Autodesk Inventor part; units mm, degrees
(part 2 of 2)
sketch "Skizze1 outline for Extrusion1" plane through (0, 0, 0) normal (0, 1, 0) x (-1, 0, 0)
  line L0 (27.3183, 0.0124) -> (29.62197, 0.0124)
  line L1 (27.3183, 0.0995) -> (27.3183, 0.0124)
  line L2 (27.2706, 0.1948) -> (27.3183, 0.0995)
  line L3 (27.223, 0.2424) -> (27.2706, 0.1948)
  line L4 (27.1278, 0.29) -> (27.223, 0.2424)
  line L5 (26.7468, 0.29) -> (27.1278, 0.29)
  line L6 (26.7468, 0.0124) -> (26.7468, 0.29)
  line L7 (11.5266, 0.0124) -> (26.7468, 0.0124)
  line L8 (10.7766, 0.7624) -> (11.5266, 0.0124)
  line L9 (9.7766, 0.7624) -> (10.7766, 0.7624)
  line L10 (9.7766, 0.0124) -> (9.7766, 0.7624)
  line L11 (8.0266, 0.0124) -> (9.7766, 0.0124)
  line L12 (6.5266, 1.5124) -> (8.0266, 0.0124)
  line L13 (1.5266, 1.5124) -> (6.5266, 1.5124)
  line L14 (1.5266, 10.9594) -> (1.5266, 1.5124)
  line L15 (16.4542, 10.9594) -> (1.5266, 10.9594)
  line L16 (26.5126, 21.0178) -> (16.4542, 10.9594)
  line L17 (31.4402, 21.0178) -> (26.5126, 21.0178)
  line L18 (31.4402, 0.0124) -> (31.4402, 21.0178)
  line L19 (30.44313, 0.0124) -> (31.4402, 0.0124)
  line L20 (30.4135, 0.0519) -> (30.44313, 0.0124)
  line L21 (30.38387, 0.0124) -> (30.4135, 0.0519)
  line L22 (29.68123, 0.0124) -> (30.38387, 0.0124)
  line L23 (29.6516, 0.0519) -> (29.68123, 0.0124)
  line L24 (29.62197, 0.0124) -> (29.6516, 0.0519)
  line L25 (20.0386, 33.4228) -> (0.125, 33.4228)
  line L26 (20.7886, 32.6728) -> (20.0386, 33.4228)
  line L27 (21.7886, 32.6728) -> (20.7886, 32.6728)
  line L28 (21.7886, 33.4228) -> (21.7886, 32.6728)
  line L29 (23.5386, 33.4228) -> (21.7886, 33.4228)
  line L30 (25.0386, 31.9228) -> (23.5386, 33.4228)
  line L31 (30.0386, 31.9228) -> (25.0386, 31.9228)
  line L32 (30.0386, 22.4758) -> (30.0386, 31.9228)
  line L33 (15.111, 22.4758) -> (30.0386, 22.4758)
  line L34 (5.0526, 12.4174) -> (15.111, 22.4758)
  line L35 (0.125, 12.4174) -> (5.0526, 12.4174)
  line L36 (0.125, 33.4228) -> (0.125, 12.4174)
  line L37 (27.2183, 36.5124) -> (29.52197, 36.5124)
  line L38 (27.2183, 36.5995) -> (27.2183, 36.5124)
  line L39 (27.1706, 36.6948) -> (27.2183, 36.5995)
  line L40 (27.123, 36.7424) -> (27.1706, 36.6948)
  line L41 (27.0278, 36.79) -> (27.123, 36.7424)
  line L42 (26.6468, 36.79) -> (27.0278, 36.79)
  line L43 (26.6468, 36.5124) -> (26.6468, 36.79)
  line L44 (11.4266, 36.5124) -> (26.6468, 36.5124)
  line L45 (10.6766, 37.2624) -> (11.4266, 36.5124)
  line L46 (9.6766, 37.2624) -> (10.6766, 37.2624)
  line L47 (9.6766, 36.5124) -> (9.6766, 37.2624)
  line L48 (7.9266, 36.5124) -> (9.6766, 36.5124)
  line L49 (6.4266, 38.0124) -> (7.9266, 36.5124)
  line L50 (1.4266, 38.0124) -> (6.4266, 38.0124)
  line L51 (1.4266, 47.4594) -> (1.4266, 38.0124)
  line L52 (16.3542, 47.4594) -> (1.4266, 47.4594)
  line L53 (26.4126, 57.5178) -> (16.3542, 47.4594)
  line L54 (31.3402, 57.5178) -> (26.4126, 57.5178)
  line L55 (31.3402, 36.5124) -> (31.3402, 57.5178)
  line L56 (30.34313, 36.5124) -> (31.3402, 36.5124)
  line L57 (30.3135, 36.5519) -> (30.34313, 36.5124)
  line L58 (30.28387, 36.5124) -> (30.3135, 36.5519)
  line L59 (29.58123, 36.5124) -> (30.28387, 36.5124)
  line L60 (29.5516, 36.5519) -> (29.58123, 36.5124)
  line L61 (29.52197, 36.5124) -> (29.5516, 36.5519)
  line L62 (19.9386, 69.9228) -> (0.025, 69.9228)
  line L63 (20.6886, 69.1728) -> (19.9386, 69.9228)
  line L64 (21.6886, 69.1728) -> (20.6886, 69.1728)
  line L65 (21.6886, 69.9228) -> (21.6886, 69.1728)
  line L66 (23.4386, 69.9228) -> (21.6886, 69.9228)
  line L67 (24.9386, 68.4228) -> (23.4386, 69.9228)
  line L68 (29.9386, 68.4228) -> (24.9386, 68.4228)
  line L69 (29.9386, 58.9758) -> (29.9386, 68.4228)
  line L70 (15.011, 58.9758) -> (29.9386, 58.9758)
  line L71 (4.9526, 48.9174) -> (15.011, 58.9758)
  line L72 (0.025, 48.9174) -> (4.9526, 48.9174)
  line L73 (0.025, 69.9228) -> (0.025, 48.9174)
  line L74 (53.0152, 69.9374) -> (33.1016, 69.9374)
  line L75 (53.7652, 69.1874) -> (53.0152, 69.9374)
  line L76 (54.7652, 69.1874) -> (53.7652, 69.1874)
  line L77 (54.7652, 69.9374) -> (54.7652, 69.1874)
  line L78 (56.5152, 69.9374) -> (54.7652, 69.9374)
  line L79 (58.0152, 68.4374) -> (56.5152, 69.9374)
  line L80 (63.0152, 68.4374) -> (58.0152, 68.4374)
  line L81 (63.0152, 58.9904) -> (63.0152, 68.4374)
  line L82 (48.0876, 58.9904) -> (63.0152, 58.9904)
  line L83 (38.0292, 48.932) -> (48.0876, 58.9904)
  line L84 (33.1016, 48.932) -> (38.0292, 48.932)
  line L85 (33.1016, 69.9374) -> (33.1016, 48.932)
  line L86 (60.2949, 36.527) -> (62.59857, 36.527)
  line L87 (60.2949, 36.6141) -> (60.2949, 36.527)
  line L88 (60.2472, 36.7094) -> (60.2949, 36.6141)
  line L89 (60.1996, 36.757) -> (60.2472, 36.7094)
  line L90 (60.1044, 36.8046) -> (60.1996, 36.757)
  line L91 (59.7234, 36.8046) -> (60.1044, 36.8046)
  line L92 (59.7234, 36.527) -> (59.7234, 36.8046)
  line L93 (44.5032, 36.527) -> (59.7234, 36.527)
  line L94 (43.7532, 37.277) -> (44.5032, 36.527)
  line L95 (42.7532, 37.277) -> (43.7532, 37.277)
  line L96 (42.7532, 36.527) -> (42.7532, 37.277)
  line L97 (41.0032, 36.527) -> (42.7532, 36.527)
  line L98 (39.5032, 38.027) -> (41.0032, 36.527)
  line L99 (34.5032, 38.027) -> (39.5032, 38.027)
  line L100 (34.5032, 47.474) -> (34.5032, 38.027)
  line L101 (49.4308, 47.474) -> (34.5032, 47.474)
  line L102 (59.4892, 57.5324) -> (49.4308, 47.474)
  line L103 (64.4168, 57.5324) -> (59.4892, 57.5324)
  line L104 (64.4168, 36.527) -> (64.4168, 57.5324)
  line L105 (63.41973, 36.527) -> (64.4168, 36.527)
  line L106 (63.3901, 36.5665) -> (63.41973, 36.527)
  line L107 (63.36047, 36.527) -> (63.3901, 36.5665)
  line L108 (62.65783, 36.527) -> (63.36047, 36.527)
  line L109 (62.6282, 36.5665) -> (62.65783, 36.527)
  line L110 (62.59857, 36.527) -> (62.6282, 36.5665)
  line L111 (53.1152, 33.4374) -> (33.2016, 33.4374)
  line L112 (53.8652, 32.6874) -> (53.1152, 33.4374)
  line L113 (54.8652, 32.6874) -> (53.8652, 32.6874)
  line L114 (54.8652, 33.4374) -> (54.8652, 32.6874)
  line L115 (56.6152, 33.4374) -> (54.8652, 33.4374)
  line L116 (58.1152, 31.9374) -> (56.6152, 33.4374)
  line L117 (63.1152, 31.9374) -> (58.1152, 31.9374)
  line L118 (63.1152, 22.4904) -> (63.1152, 31.9374)
  line L119 (48.1876, 22.4904) -> (63.1152, 22.4904)
  line L120 (38.1292, 12.432) -> (48.1876, 22.4904)
  line L121 (33.2016, 12.432) -> (38.1292, 12.432)
  line L122 (33.2016, 33.4374) -> (33.2016, 12.432)
  line L123 (60.3949, 0.027) -> (62.69857, 0.027)
  line L124 (60.3949, 0.1141) -> (60.3949, 0.027)
  line L125 (60.3472, 0.2094) -> (60.3949, 0.1141)
  line L126 (60.2996, 0.257) -> (60.3472, 0.2094)
  line L127 (60.2044, 0.3046) -> (60.2996, 0.257)
  line L128 (59.8234, 0.3046) -> (60.2044, 0.3046)
  line L129 (59.8234, 0.027) -> (59.8234, 0.3046)
  line L130 (44.6032, 0.027) -> (59.8234, 0.027)
  line L131 (43.8532, 0.777) -> (44.6032, 0.027)
  line L132 (42.8532, 0.777) -> (43.8532, 0.777)
  line L133 (42.8532, 0.027) -> (42.8532, 0.777)
  line L134 (41.1032, 0.027) -> (42.8532, 0.027)
  line L135 (39.6032, 1.527) -> (41.1032, 0.027)
  line L136 (34.6032, 1.527) -> (39.6032, 1.527)
  line L137 (34.6032, 10.974) -> (34.6032, 1.527)
  line L138 (49.5308, 10.974) -> (34.6032, 10.974)
  line L139 (59.5892, 21.0324) -> (49.5308, 10.974)
  line L140 (64.5168, 21.0324) -> (59.5892, 21.0324)
  line L141 (64.5168, 0.027) -> (64.5168, 21.0324)
  line L142 (63.51973, 0.027) -> (64.5168, 0.027)
  line L143 (63.4901, 0.0665) -> (63.51973, 0.027)
  line L144 (63.46047, 0.027) -> (63.4901, 0.0665)
  line L145 (62.75783, 0.027) -> (63.46047, 0.027)
  line L146 (62.7282, 0.0665) -> (62.75783, 0.027)
  line L147 (62.69857, 0.027) -> (62.7282, 0.0665)
  line L148 (94.0699, 0.027) -> (96.37357, 0.027)
  line L149 (94.0699, 0.1141) -> (94.0699, 0.027)
  line L150 (94.0222, 0.2094) -> (94.0699, 0.1141)
  line L151 (93.9746, 0.257) -> (94.0222, 0.2094)
  line L152 (93.8794, 0.3046) -> (93.9746, 0.257)
  line L153 (93.4984, 0.3046) -> (93.8794, 0.3046)
  line L154 (93.4984, 0.027) -> (93.4984, 0.3046)
  line L155 (78.2782, 0.027) -> (93.4984, 0.027)
  line L156 (77.5282, 0.777) -> (78.2782, 0.027)
  line L157 (76.5282, 0.777) -> (77.5282, 0.777)
  line L158 (76.5282, 0.027) -> (76.5282, 0.777)
  line L159 (74.7782, 0.027) -> (76.5282, 0.027)
  line L160 (73.2782, 1.527) -> (74.7782, 0.027)
  line L161 (68.2782, 1.527) -> (73.2782, 1.527)
  line L162 (68.2782, 10.974) -> (68.2782, 1.527)
  line L163 (83.2058, 10.974) -> (68.2782, 10.974)
  line L164 (93.2642, 21.0324) -> (83.2058, 10.974)
  line L165 (98.1918, 21.0324) -> (93.2642, 21.0324)
  line L166 (98.1918, 0.027) -> (98.1918, 21.0324)
  line L167 (97.19473, 0.027) -> (98.1918, 0.027)
  line L168 (97.1651, 0.0665) -> (97.19473, 0.027)
  line L169 (97.13547, 0.027) -> (97.1651, 0.0665)
  line L170 (96.43283, 0.027) -> (97.13547, 0.027)
  line L171 (96.4032, 0.0665) -> (96.43283, 0.027)
  line L172 (96.37357, 0.027) -> (96.4032, 0.0665)
  line L173 (86.7902, 33.4374) -> (66.8766, 33.4374)
  line L174 (87.5402, 32.6874) -> (86.7902, 33.4374)
  line L175 (88.5402, 32.6874) -> (87.5402, 32.6874)
  line L176 (88.5402, 33.4374) -> (88.5402, 32.6874)
  line L177 (90.2902, 33.4374) -> (88.5402, 33.4374)
  line L178 (91.7902, 31.9374) -> (90.2902, 33.4374)
  line L179 (96.7902, 31.9374) -> (91.7902, 31.9374)
  line L180 (96.7902, 22.4904) -> (96.7902, 31.9374)
  line L181 (81.8626, 22.4904) -> (96.7902, 22.4904)
  line L182 (71.8042, 12.432) -> (81.8626, 22.4904)
  line L183 (66.8766, 12.432) -> (71.8042, 12.432)
  line L184 (66.8766, 33.4374) -> (66.8766, 12.432)
  line L185 (93.9699, 36.527) -> (96.27357, 36.527)
  line L186 (93.9699, 36.6141) -> (93.9699, 36.527)
  line L187 (93.9222, 36.7094) -> (93.9699, 36.6141)
  line L188 (93.8746, 36.757) -> (93.9222, 36.7094)
  line L189 (93.7794, 36.8046) -> (93.8746, 36.757)
  line L190 (93.3984, 36.8046) -> (93.7794, 36.8046)
  line L191 (93.3984, 36.527) -> (93.3984, 36.8046)
  line L192 (78.1782, 36.527) -> (93.3984, 36.527)
  line L193 (77.4282, 37.277) -> (78.1782, 36.527)
  line L194 (76.4282, 37.277) -> (77.4282, 37.277)
  line L195 (76.4282, 36.527) -> (76.4282, 37.277)
  line L196 (74.6782, 36.527) -> (76.4282, 36.527)
  line L197 (73.1782, 38.027) -> (74.6782, 36.527)
  line L198 (68.1782, 38.027) -> (73.1782, 38.027)
  line L199 (68.1782, 47.474) -> (68.1782, 38.027)
  line L200 (83.1058, 47.474) -> (68.1782, 47.474)
  line L201 (93.1642, 57.5324) -> (83.1058, 47.474)
  line L202 (98.0918, 57.5324) -> (93.1642, 57.5324)
  line L203 (98.0918, 36.527) -> (98.0918, 57.5324)
  line L204 (97.09473, 36.527) -> (98.0918, 36.527)
  line L205 (97.0651, 36.5665) -> (97.09473, 36.527)
  line L206 (97.03547, 36.527) -> (97.0651, 36.5665)
  line L207 (96.33283, 36.527) -> (97.03547, 36.527)
  line L208 (96.3032, 36.5665) -> (96.33283, 36.527)
  line L209 (96.27357, 36.527) -> (96.3032, 36.5665)
  line L210 (86.6902, 69.9374) -> (66.7766, 69.9374)
  line L211 (87.4402, 69.1874) -> (86.6902, 69.9374)
  line L212 (88.4402, 69.1874) -> (87.4402, 69.1874)
  line L213 (88.4402, 69.9374) -> (88.4402, 69.1874)
  line L214 (90.1902, 69.9374) -> (88.4402, 69.9374)
  line L215 (91.6902, 68.4374) -> (90.1902, 69.9374)
  line L216 (96.6902, 68.4374) -> (91.6902, 68.4374)
  line L217 (96.6902, 58.9904) -> (96.6902, 68.4374)
  line L218 (81.7626, 58.9904) -> (96.6902, 58.9904)
  line L219 (71.7042, 48.932) -> (81.7626, 58.9904)
  line L220 (66.7766, 48.932) -> (71.7042, 48.932)
  line L221 (66.7766, 69.9374) -> (66.7766, 48.932)
  line L222 (119.767, 69.952) -> (99.8532, 69.952)
  line L223 (120.517, 69.202) -> (119.767, 69.952)
  line L224 (121.517, 69.202) -> (120.517, 69.202)
  line L225 (121.517, 69.952) -> (121.517, 69.202)
  line L226 (123.267, 69.952) -> (121.517, 69.952)
  line L227 (124.767, 68.452) -> (123.267, 69.952)
  line L228 (129.767, 68.452) -> (124.767, 68.452)
  line L229 (129.767, 59.005) -> (129.767, 68.452)
  line L230 (114.839, 59.005) -> (129.767, 59.005)
  line L231 (104.781, 48.9466) -> (114.839, 59.005)
  line L232 (99.8532, 48.9466) -> (104.781, 48.9466)
  line L233 (99.8532, 69.952) -> (99.8532, 48.9466)
  line L234 (127.046, 36.5416) -> (129.350349, 36.5416)
  line L235 (127.046, 36.6287) -> (127.046, 36.5416)
  line L236 (126.999, 36.724) -> (127.046, 36.6287)
  line L237 (126.951, 36.7716) -> (126.999, 36.724)
  line L238 (126.856, 36.8192) -> (126.951, 36.7716)
  line L239 (126.475, 36.8192) -> (126.856, 36.8192)
  line L240 (126.475, 36.5416) -> (126.475, 36.8192)
  line L241 (111.255, 36.5416) -> (126.475, 36.5416)
  line L242 (110.505, 37.2916) -> (111.255, 36.5416)
  line L243 (109.505, 37.2916) -> (110.505, 37.2916)
  line L244 (109.505, 36.5416) -> (109.505, 37.2916)
  line L245 (107.755, 36.5416) -> (109.505, 36.5416)
  line L246 (106.255, 38.0416) -> (107.755, 36.5416)
  line L247 (101.255, 38.0416) -> (106.255, 38.0416)
  line L248 (101.255, 47.4886) -> (101.255, 38.0416)
  line L249 (116.182, 47.4886) -> (101.255, 47.4886)
  line L250 (126.241, 57.547) -> (116.182, 47.4886)
  line L251 (131.168, 57.547) -> (126.241, 57.547)
  line L252 (131.168, 36.5416) -> (131.168, 57.547)
  line L253 (130.171651, 36.5416) -> (131.168, 36.5416)
  line L254 (130.142, 36.5811) -> (130.171651, 36.5416)
  line L255 (130.112349, 36.5416) -> (130.142, 36.5811)
  line L256 (129.409651, 36.5416) -> (130.112349, 36.5416)
  line L257 (129.38, 36.5811) -> (129.409651, 36.5416)
  line L258 (129.350349, 36.5416) -> (129.38, 36.5811)
  line L259 (119.867, 33.452) -> (99.9532, 33.452)
  line L260 (120.617, 32.702) -> (119.867, 33.452)
  line L261 (121.617, 32.702) -> (120.617, 32.702)
  line L262 (121.617, 33.452) -> (121.617, 32.702)
  line L263 (123.367, 33.452) -> (121.617, 33.452)
  line L264 (124.867, 31.952) -> (123.367, 33.452)
  line L265 (129.867, 31.952) -> (124.867, 31.952)
  line L266 (129.867, 22.505) -> (129.867, 31.952)
  line L267 (114.939, 22.505) -> (129.867, 22.505)
  line L268 (104.881, 12.4466) -> (114.939, 22.505)
  line L269 (99.9532, 12.4466) -> (104.881, 12.4466)
  line L270 (99.9532, 33.452) -> (99.9532, 12.4466)
  line L271 (127.147, 0.0416) -> (129.450349, 0.0416)
  line L272 (127.147, 0.1287) -> (127.147, 0.0416)
  line L273 (127.099, 0.224) -> (127.147, 0.1287)
  line L274 (127.051, 0.2716) -> (127.099, 0.224)
  line L275 (126.956, 0.3192) -> (127.051, 0.2716)
  line L276 (126.575, 0.3192) -> (126.956, 0.3192)
  line L277 (126.575, 0.0416) -> (126.575, 0.3192)
  line L278 (111.355, 0.0416) -> (126.575, 0.0416)
  line L279 (110.605, 0.7916) -> (111.355, 0.0416)
  line L280 (109.605, 0.7916) -> (110.605, 0.7916)
  line L281 (109.605, 0.0416) -> (109.605, 0.7916)
  line L282 (107.855, 0.0416) -> (109.605, 0.0416)
  line L283 (106.355, 1.5416) -> (107.855, 0.0416)
  line L284 (101.355, 1.5416) -> (106.355, 1.5416)
  line L285 (101.355, 10.9886) -> (101.355, 1.5416)
  line L286 (116.282, 10.9886) -> (101.355, 10.9886)
  line L287 (126.341, 21.047) -> (116.282, 10.9886)
  line L288 (131.268, 21.047) -> (126.341, 21.047)
  line L289 (131.268, 0.0416) -> (131.268, 21.047)
  line L290 (130.271651, 0.0416) -> (131.268, 0.0416)
  line L291 (130.242, 0.0811) -> (130.271651, 0.0416)
  line L292 (130.212349, 0.0416) -> (130.242, 0.0811)
  line L293 (129.509651, 0.0416) -> (130.212349, 0.0416)
  line L294 (129.48, 0.0811) -> (129.509651, 0.0416)
  line L295 (129.450349, 0.0416) -> (129.48, 0.0811)
extrude "Extrusion1" add sketch "Skizze1 outline for Extrusion1" along normal blind 0.6
